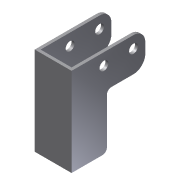
# Autodesk Inventor part: CounterWeight
Saved by Autodesk Inventor 2011 SP1 (Build 150282100, 282)
## iProperties
Created: 2012-10-16
Part Number: CounterWeight
Document SubType Name: Modeling
Designer: arihon
Density: 1 g/cm^3
Author: arihon
Autodesk Inventor part; units mm, degrees
ref_plane "YZ Plane" through (0, 0, 0) normal (1, 0, 0) x (0, 1, 0)
ref_plane "XZ Plane" through (0, 0, 0) normal (0, 1, 0) x (-1, 0, 0)
ref_plane "XY Plane" through (0, 0, 0) normal (0, 0, 1) x (1, 0, 0)
sketch "スケッチ1" plane through (0, 0, 0) normal (0, 0, 1) x (1, 0, 0)
  line L0 (-12.5, 25) -> (12.5, 25)
  line L1 (12.5, 25) -> (12.5, -25)
  line L2 (12.5, -25) -> (-12.5, -25)
  line L3 (-12.5, -25) -> (-12.5, 25)
  line L4 (-10.5, 25) -> (10.5, 25)
  line L5 (10.5, 25) -> (10.5, -23)
  line L6 (10.5, -23) -> (-10.5, -23)
  line L7 (-10.5, -23) -> (-10.5, 25)
  point P0 (0, 0)
  dimension "d0" = 25
  dimension "d1" = 50
  dimension "d2" = 25
  dimension "d3" = 12.5
  dimension "d4" = 2
  dimension "d5" = 2
  dimension "d6" = 2
  constraints: 16 end point, 4 parallel, 2 horizontal, 2 perpendicular, 1 point on line
  measures "d0" distance of L0.start L0.end
  measures "d1" distance of L2.end L0.start
  measures "d2" distance from line of L0 point (0, 0)
  measures "d3" distance from line of L3 point (0, 0)
  measures "d4" distance between parallel lines of L3 L7
  measures "d5" distance between parallel lines of L1 L5
  measures "d6" distance between parallel lines of L2 L6
extrude "押し出し1" add sketch "スケッチ1" along normal blind 60 contours L0 L7 L6 L5 L1 L2 L3
sketch "スケッチ2" plane through (12.5, -25, 0) normal (1, 0, 0) x (0, 0, -1)
  line L0 (0, 50) -> (-60, 50) projected
  line L1 (-30, 50) -> (-30, 0)
  line L2 (0, 0) -> (-60, 0) projected
  line L3 (-60, 50) -> (-60, 0) projected
  point P0 (0, 25)
  point P1 (-52, 42)
  point P2 (-52, 22)
  dimension "d12" = 8
  dimension "d76" = 8
  dimension "d85" = 8
  dimension "d86" = 20
  constraints: 2 end point, 2 midpoint
  measures "d12" distance from line of L0 point (-52, 42)
  measures "d76" distance from line of L3 point (-52, 42)
  measures "d85" distance from line of point (-52, 22) L3
  measures "d86" distance of point (-52, 22) point (-52, 42)
hole "Hole1" at (12.5, 17, 52) at (12.5, -3, 52) direction (-1, 0, 0) diameter 6 end through all
sketch "スケッチ9" plane through (12.5, -25, 0) normal (1, 0, 0) x (0, 0, -1)
  circle A0 centre (-52, 22) radius 3 projected
  line L0 (0, 50) -> (-37, 50)
  line L1 (-37, 50) -> (-37, 24)
  line L2 (-37, 24) -> (0, 24)
  line L3 (0, 24) -> (0, 50)
  line L4 (0, 2) -> (-60, 2) projected
  point P0 (0, 25)
  dimension "d77" = 15
  dimension "d78" = 22
  constraints: 8 end point, 2 parallel, 1 horizontal, 1 perpendicular
  measures "d77" distance from line of L1 A0.centre
  measures "d78" distance between parallel lines of L4 L2
extrude "押し出し5" cut sketch "スケッチ9" against normal through all contours L3 L2 L1 L0
fillet "フィレット5" radius 3 2 edges at (11.5, -1, 37) (-11.5, -1, 37)
fillet "フィレット6" radius 8 4 edges at (-11.5, 25, 60) (11.5, 25, 60) (11.5, 25, 37) (-11.5, 25, 37)
fillet "フィレット7" radius 3 2 edges at (11.5, -1, 0) (-11.5, -1, 0)
equation "\"d1\" = 2 * d0"
equation "\"d2\" = 0.5 * d1"
equation "\"d3\" = 0.5 * d0"
equation "\"d4\" = d5"
equation "\"d6\" = d5"
equation "\"d12\" = d11"
equation "\"d76\" = d11"
equation "\"d85\" = d76"
equation "\"d11\" = 8"
